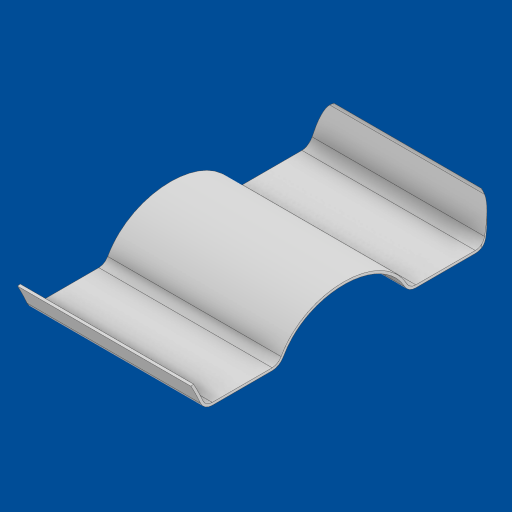
# Autodesk Inventor part: cover_bottom
Saved by Autodesk Inventor 2023.1 (Build 271208000, 208)
## iProperties
Created: 2023-06-05
Part Number: cover_bottom
Material: Generic
Document SubType Name: Modeling
Designer: nara atthama
Density: 1 g/cm^3
Appearance: Default
Author: nara atthama
Autodesk Inventor part; units mm, degrees
ref_plane "YZ Plane" through (0, 0, 0) normal (1, 0, 0) x (0, 1, 0)
ref_plane "XZ Plane" through (0, 0, 0) normal (0, 1, 0) x (-1, 0, 0)
ref_plane "XY Plane" through (0, 0, 0) normal (0, 0, 1) x (1, 0, 0)
derived "top_case.ipt"
sketch "Sketch13" plane through (0, 70, 0) normal (0, 1, 0) x (1, 0, 0)
  arc A0 (-30, 60) -> (-35, 55) centre (-30, 55) ccw
  line L0 (-35, 55) -> (-35, -60)
  line L1 (-35, -60) -> (-34, -60)
  line L2 (-34, -60) -> (-34, 54)
  arc A1 (-29, 59) -> (-34, 54) centre (-29, 54) ccw
  line L3 (-29, 59) -> (29, 59)
  arc A2 (34, 54) -> (29, 59) centre (29, 54) ccw
  line L4 (34, 54) -> (34, -60)
  line L5 (34, -60) -> (35, -60)
  line L6 (35, -60) -> (35, 55)
  arc A3 (35, 55) -> (30, 60) centre (30, 55) ccw
  line L7 (30, 60) -> (-30, 60)
  point P0 (0, 0)
sketch "Sketch12" plane through (35, 30, 60) normal (1, 0, 0) x (0, 0, -1)
  arc A0 (119.7605, -15.7057) -> (120, -14.1768) centre (115, -14.1768) ccw projected
  line L0 (120, -14.1768) -> (120, 40) projected
  line L1 (0, 40) -> (120, 40) projected
  line L2 (0, 0) -> (0, 40) projected
  line L3 (0, -19.3605) -> (0, 0) projected
  arc A1 (3.7459, -27.0066) -> (0, -19.3605) centre (-87.8477, -67.1391) ccw projected
  arc A2 (3.7459, -27.0066) -> (8.3256, -30) centre (8.3256, -25) ccw projected
  line L4 (8.3256, -30) -> (31.8504, -30) projected
  line L5 (88.1797, -30) -> (111.524, -30) projected
  arc A3 (111.524, -30) -> (116.2845, -26.5289) centre (111.524, -25) ccw projected
  line L6 (116.2845, -26.5289) -> (119.7605, -15.7057) projected
  circle A4 centre (95.5, -24) radius 0.9 projected
  circle A5 centre (100, -24) radius 1.75 projected
  circle A6 centre (104.5, -24) radius 0.9 projected
  circle A7 centre (20, -24) radius 1.75 projected
  spline S0 degree 3 poles (36.2216, -27.4275) (35.9055, -27.9967) (35.4813, -28.4987) (34.5327, -29.2571) (34.0364, -29.532) (32.9731, -29.9048) (32.4138, -30) (31.8504, -30) knots 0 0 0 0 0.195322 0.195322 0.364334 0.364334 0.533346 0.533346 0.533346 0.533346 projected
  spline S1 degree 3 poles (36.2216, -27.4275) (37.1467, -25.7615) (38.2802, -24.2255) (41.6483, -20.7162) (44.0653, -19.0238) (49.904, -16.2193) (53.4, -15.3109) (61.0863, -14.5978) (65.3697, -15.0119) (72.7146, -17.2747) (75.8948, -18.8974) (79.9949, -22.3069) (81.2512, -23.6277) (82.8687, -25.8385) (83.3587, -26.6082) (83.7968, -27.4063) knots 0.286984 0.286984 0.286984 0.286984 0.865656 0.865656 1.747886 1.747886 2.81107 2.81107 4.064213 4.064213 5.119563 5.119563 5.66782 5.66782 5.943286 5.943286 5.943286 5.943286 projected
  spline S2 degree 3 poles (88.1797, -30) (87.5287, -30) (86.8838, -29.8728) (85.7565, -29.4102) (85.2721, -29.107) (84.4257, -28.351) (84.0699, -27.9037) (83.7968, -27.4063) knots 0 0 0 0 0.195322 0.195322 0.365552 0.365552 0.535783 0.535783 0.535783 0.535783 projected
  line L7 (31.8504, -29) -> (8.3256, -29)
  arc A8 (4.6619, -26.6053) -> (8.3256, -29) centre (8.3256, -25) ccw
  arc A9 (4.6619, -26.6053) -> (1, -19.1069) centre (-87.8477, -67.1391) ccw
  line L8 (1, -19.1069) -> (1, 0) construction
  line L9 (1, 0) -> (1, 39)
  line L10 (1, 39) -> (119, 39)
  line L11 (119, 39) -> (119, -14.1768) construction
  arc A10 (118.8084, -15.3999) -> (119, -14.1768) centre (115, -14.1768) ccw
  line L12 (118.8084, -15.3999) -> (115.3324, -26.2231)
  arc A11 (111.524, -29) -> (115.3324, -26.2231) centre (111.524, -25) ccw
  line L13 (111.524, -29) -> (88.1797, -29)
  line L14 (1, -19.1069) -> (0, -19.3605)
  line L15 (119, -14.1768) -> (120, -14.1768)
  spline S3 degree 5 poles (84.6734, -26.925) (83.2606, -24.3513) (81.4167, -22.0101) (79.2006, -20.0102) (74.2903, -16.7212) (68.7008, -14.7966) (65.822, -14.1651) (59.9731, -13.5279) (54.1238, -14.156) (51.2444, -14.7854) (45.6688, -16.7212) (40.7867, -20.035) (38.5935, -22.0462) (36.7681, -24.3836) (35.3474, -26.942) knots 0 0 0 0 0 0 0.250718 0.250718 0.250718 0.500464 0.500464 0.500464 0.750104 0.750104 0.750104 1 1 1 1 1 1
  spline S4 degree 4 poles (35.3474, -26.942) (34.8316, -27.8715) (33.9815, -28.6212) (32.9134, -29.0004) (31.8504, -29) knots 0 0 0 0 0 1 1 1 1 1
  spline S5 degree 4 poles (88.1797, -29) (87.1119, -29.0004) (86.0388, -28.6177) (85.1869, -27.8613) (84.6734, -26.925) knots 0 0 0 0 0 1 1 1 1 1
  point P0 (60, -30)
  dimension "d1" = 1
  constraints: 18 end point, 8 point on circle, 4 centre point, 2 parallel, 1 horizontal, 19 other
extrude "Extrusion1" add sketch "Sketch12" against normal blind 70 contours L6 A3 L5 S2 S1 S0 L4 A2 A1 L14 A9 A8 L7 S4 S3 S5 L13 A11 L12 A10 L15 A0
split body "Split1" sketch "Sketch13" result one side removed curves L1 L2 A1 L3 A2 L4 L5 removed pieces at (-9.6667, 13.2253, -59.1)
body "Solid1"
